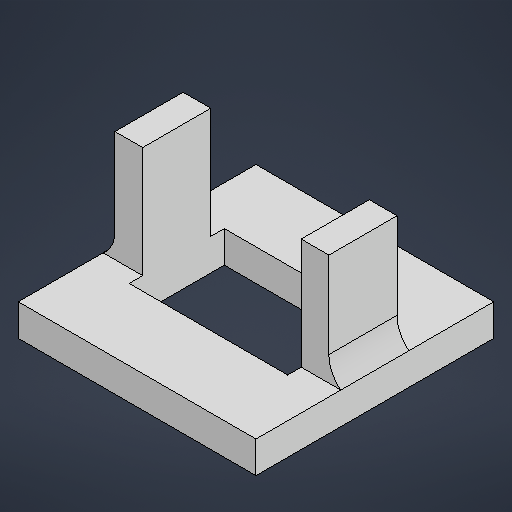
# Autodesk Inventor part: LRA_case3
Saved by Autodesk Inventor 2026 (Build 300175050, 175E)
## iProperties
Created: 2025-09-05
Part Number: LRA_case3
Material: 一般
Document SubType Name: Modeling
Designer: ka0n7
Density: 1 g/cm^3
Appearance: 既定
Author: ka0n7
Autodesk Inventor part; units mm, degrees
ref_plane "YZ Plane" through (0, 0, 0) normal (1, 0, 0) x (0, 1, 0)
ref_plane "XZ Plane" through (0, 0, 0) normal (0, 1, 0) x (-1, 0, 0)
ref_plane "XY Plane" through (0, 0, 0) normal (0, 0, 1) x (1, 0, 0)
sketch "スケッチ1" plane through (0, 0, 0) normal (0, 1, 0) x (-1, 0, 0)
  line L0 (7.5, 7.5) -> (-7.5, 7.5)
  line L1 (-7.5, 7.5) -> (-7.5, -7.5)
  line L2 (-7.5, -7.5) -> (7.5, -7.5)
  line L3 (7.5, -7.5) -> (7.5, 7.5)
  line L4 (7.5, 7.5) -> (-7.5, -7.5) construction
  line L5 (-7.5, 7.5) -> (7.5, -7.5) construction
  line L6 (5, 3) -> (-5, 3)
  line L7 (-5, 3) -> (-5, -3)
  line L8 (-5, -3) -> (5, -3)
  line L9 (5, -3) -> (5, 3)
  line L10 (5, 3) -> (-5, -3) construction
  line L11 (-5, 3) -> (5, -3) construction
  point P0 (0, 0)
  dimension "d0" = 15
  dimension "d1" = 15
  dimension "d2" = 10
  dimension "d3" = 6
  constraints: 24 end point, 4 midpoint, 4 parallel, 2 horizontal, 2 perpendicular
  measures "d0" distance of L2.end L1.end
  measures "d1" distance of L2.end L0.start
  measures "d2" distance of L8.end L7.end
  measures "d3" distance of L8.end L6.start
extrude "押し出し1" add sketch "スケッチ1" along normal blind 2
sketch "スケッチ2" plane through (0, 2, 0) normal (0, 1, 0) x (1, 0, 0)
  line L0 (-6.75, 2.15) -> (6.75, 2.15)
  line L1 (6.75, 2.15) -> (6.75, -2.15)
  line L2 (6.75, -2.15) -> (-6.75, -2.15)
  line L3 (-6.75, -2.15) -> (-6.75, 2.15)
  line L4 (-6.75, 2.15) -> (6.75, -2.15) construction
  line L5 (6.75, 2.15) -> (-6.75, -2.15) construction
  line L6 (-5, -3) -> (-5, 3) projected
  line L7 (-5, 2.15) -> (-5, -2.15)
  line L8 (5, 3) -> (5, -3) projected
  line L9 (5, 2.15) -> (5, -2.15)
  point P0 (0, 0)
  dimension "d8" = 13.5
  dimension "d9" = 4.3
  constraints: 16 end point, 8 point on line, 2 midpoint, 2 parallel, 1 horizontal, 1 perpendicular
  measures "d8" distance of L1.end L2.end
  measures "d9" distance of L0.end L1.end
extrude "押し出し2" add sketch "スケッチ2" along normal blind 7 contours L0 L6 L2 L3 | L0 L1 L2 L8
fillet "フィレット1" radius 2 2 edges at (6.75, 2, 0) (-6.75, 2, 0)
